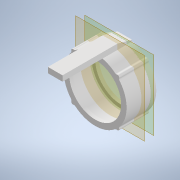
# Autodesk Inventor part: inner_part
Saved by Autodesk Inventor 2021 (Build 250183000, 183)
## iProperties
Created: 2022-07-01
Part Number: inner_part
Material: Типовые
Document SubType Name: Modeling
Designer: termi
Density: 1 g/cm^3
Appearance: По умолчанию
Mass: 408.389 g
Surface Area: 1227.86 cm^2
Volume: 408.389 cm^3
Author: termi
Autodesk Inventor part; units mm, degrees
ref_plane "YZ Plane" through (0, 0, 0) normal (1, 0, 0) x (0, 1, 0)
ref_plane "XZ Plane" through (0, 0, 0) normal (0, 1, 0) x (-1, 0, 0)
ref_plane "XY Plane" through (0, 0, 0) normal (0, 0, 1) x (1, 0, 0)
sketch "Эскиз1" plane through (0, 0, 0) normal (0, 1, 0) x (-1, 0, 0)
  line L0 (-79.4, 472) -> (79.4, 472) projected
  line L1 (71, 472) -> (81, 472)
  line L2 (81, 472) -> (81, 411)
  line L3 (81, 411) -> (71, 411)
  line L4 (71, 411) -> (71, 401)
  line L5 (71, 401) -> (86, 401)
  line L6 (86, 401) -> (86, 482)
  line L7 (86, 482) -> (71, 482)
  line L8 (71, 482) -> (71, 472)
  line L9 (0, 518.459) -> (0, 326.4239)
  point P0 (0, 0)
  dimension "d0" = 5
  dimension "d1" = 10
  dimension "d3" = 61
  dimension "d4" = 142
  dimension "d5" = 162
  constraints: 18 end point, 6 perpendicular, 4 point on line, 2 vertical, 1 collinear
  measures "d0" distance between parallel lines of L6 L2
  measures "d1" distance between parallel lines of L0 L7
  measures "d3" distance between parallel lines of L3 L1
  measures "d4" diameter of L8 L9
  measures "d5" diameter of L2 L9
revolve "Вращение1" add sketch "Эскиз1" angle 360 about axis through (0, 0, 518.459) along (0, 0, -1)
ref_plane "РабПлоскость1" through (0, 0, 441.5) normal (0, 0, 1) x (1, 0, 0)
ref_plane "РабПлоскость4" through (0, 0, 482) normal (0, 0, 1) x (1, 0, 0)
sketch "Эскиз2" plane through (0, 0, 482) normal (0, 0, 1) x (1, 0, 0)
  circle A0 centre (0, 0) radius 86 projected
  line L0 (-15, 72.7645) -> (15, 72.7645)
  line L1 (15, 72.7645) -> (15, 82.7645)
  line L2 (15, 82.7645) -> (-15, 82.7645)
  line L3 (-15, 82.7645) -> (-15, 72.7645)
  circle A1 centre (0, 0) radius 86 projected
  point P0 (0, 0)
  point P1 (0, 82.7645)
  dimension "d7" = 30
  dimension "d8" = 10
  constraints: 8 end point, 2 parallel, 1 horizontal, 1 midpoint, 1 perpendicular, 1 vertical alignment, 1 other
  measures "d7" distance between parallel lines of L1 L3
  measures "d8" distance from line of L0.end L2
extrude "Выдавливание1" add sketch "Эскиз2" along normal blind 150 contours L3 L2 L1 L0
sketch "Эскиз3" plane through (0, 0, 482) normal (0, 0, 1) x (1, 0, 0)
  line L0 (0, 0) -> (101.7015, 101.7015) construction
  line L1 (0, 0) -> (143.8277, 0) construction
  circle A0 centre (0, 0) radius 86 projected
  arc A1 (64.2424, 57.1744) -> (57.1744, 64.2424) centre (60.8112, 60.8112) ccw
  point P0 (20, 83.6421)
  point P1 (-20, 83.6421)
  dimension "d12" = 45
  dimension "d13" = 10
  constraints: 5 point on circle, 4 end point, 1 centre point, 1 equal length, 1 horizontal, 1 point on line
  measures "d12" angle of L1 L0
  measures "d13" diameter of A1
extrude "Выдавливание2" add sketch "Эскиз3" against normal up to surface (81 mm away) contours A0 A1
fillet "Сопряжение1" radius 5 2 edges at (57.1744, 64.2424, 441.5) (64.2424, 57.1744, 441.5)
ref_plane "РабПлоскость2" through (20, 87.7902, 416) normal (0, 0, -1) x (-1, 0, 0)
sketch "Эскиз4" plane through (20, 69.1605, 401) normal (0, 0, -1) x (-1, 0, 0)
  arc A0 (-39.2789, -3.5899) -> (-45.5706, -9.8816) centre (-40.8112, -8.3493) ccw projected
  point P0 (20, -69.1605)
hole "Отверстие1" at (60.8112, 60.8112, 401) direction (0, 0, 1) diameter 4 depth 37.75 tip angle 118 counterbore diameter 8 counterbore depth 4
pattern_circular "Круговой массив1" count 4 over 360 about axis through (0, 0, 441.5) along (0, 0, -1) of "Выдавливание2", "Отверстие1", "Сопряжение1"
split body "Разделение2" result two bodies by plane through (20, 87.7902, 416) normal (0, 0, -1) first body at (0, 75.8383, 401.5)
sketch "Эскиз5" plane through (-15, 82.7645, 632) normal (0, 1, 0) x (1, 0, 0)
  arc A0 (0, 15) -> (30, 15) centre (15, 15) ccw
  line L0 (0, 150) -> (0, 0) projected
  line L1 (30, 0) -> (0, 0) projected
  line L2 (30, 150) -> (30, 0) projected
  circle A1 centre (15, 15) radius 10
  point P0 (15, 632)
  point P1 (40, 150)
  point P2 (15, 0)
  dimension "d30" = 20
  constraints: 2 centre point, 2 point on circle, 2 tangent, 1 coincident, 1 point on line, 3 other
  measures "d30" diameter of A1
extrude "Выдавливание3" cut sketch "Эскиз5" against normal blind 20.75 bodies 3
